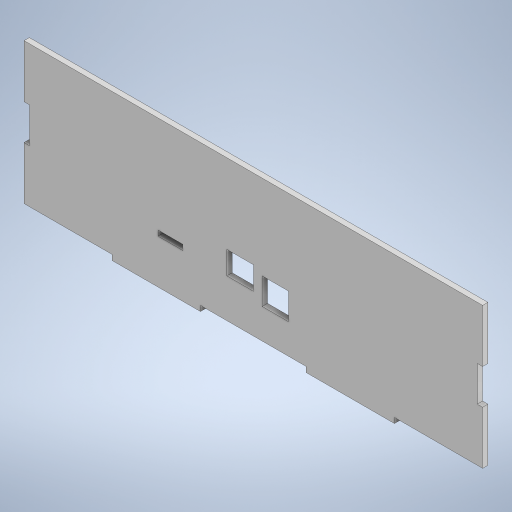
# Autodesk Inventor part: Depan
Saved by Autodesk Inventor 2024 (Build 280153000, 153)
## iProperties
Created: 2023-08-09
Part Number: Depan
Material: Generic
Document SubType Name: Modeling
Designer: Asus
Density: 1 g/cm^3
Appearance: Default
Author: Asus
Autodesk Inventor part; units mm, degrees
ref_plane "YZ Plane" through (0, 0, 0) normal (1, 0, 0) x (0, 1, 0)
ref_plane "XZ Plane" through (0, 0, 0) normal (0, 1, 0) x (-1, 0, 0)
ref_plane "XY Plane" through (0, 0, 0) normal (0, 0, 1) x (1, 0, 0)
sketch "Sketch1" plane through (0, 0, 0) normal (0, 0, 1) x (1, 0, 0)
  line L0 (0, 0) -> (0, 3) construction
  line L1 (0, 3) -> (50, 3)
  line L2 (50, 3) -> (50, 0)
  line L3 (50, 0) -> (100, 0)
  line L4 (100, 0) -> (100, 3)
  line L5 (100, 3) -> (160, 3)
  line L6 (160, 3) -> (160, 0)
  line L7 (160, 0) -> (210, 0)
  line L8 (210, 0) -> (210, 3)
  line L9 (210, 3) -> (260, 3)
  line L10 (260, 3) -> (260, 33)
  line L11 (260, 33) -> (257, 33)
  line L12 (257, 33) -> (257, 53)
  line L13 (257, 53) -> (260, 53)
  line L14 (260, 53) -> (260, 83)
  line L15 (0, 83) -> (0, 53)
  line L16 (0, 53) -> (3, 53)
  line L17 (3, 53) -> (3, 33)
  line L18 (3, 33) -> (0, 33)
  line L19 (0, 33) -> (0, 3)
  line L20 (260, 0) -> (260, 25) construction
  line L21 (260, 25) -> (260, 28) construction
  line L22 (260, 28) -> (90, 28) construction
  line L23 (90, 28) -> (90, 25)
  line L24 (90, 25) -> (76, 25)
  line L25 (76, 25) -> (76, 28)
  line L26 (76, 28) -> (90, 28)
  line L27 (90, 28) -> (135, 28) construction
  line L28 (135, 28) -> (135, 0) construction
  line L29 (135, 0) -> (135, 20) construction
  line L30 (135, 20) -> (150, 20) construction
  line L31 (135, 20) -> (135, 35)
  line L32 (135, 35) -> (150, 35)
  line L33 (150, 35) -> (150, 20)
  line L34 (135, 20) -> (150, 20)
  line L35 (90, 28) -> (117, 28) construction
  line L36 (117, 28) -> (130, 28) construction
  line L37 (130, 28) -> (130, 0) construction
  line L38 (130, 0) -> (130, 25) construction
  line L39 (130, 25) -> (130, 38) construction
  line L40 (130, 25) -> (115, 25)
  line L41 (115, 25) -> (115, 38)
  line L42 (115, 38) -> (130, 38)
  line L43 (130, 25) -> (130, 38)
  line L44 (0, 83) -> (260, 83)
  point P0 (0, 18)
  dimension "d0" = 3
  dimension "d2" = 50
  dimension "d3" = 60
  dimension "d4" = 50
  dimension "d5" = 50
  dimension "d6" = 30
  dimension "d7" = 3
  dimension "d8" = 20
  dimension "d9" = 30
  dimension "d10" = 30
  dimension "d11" = 3
  dimension "d12" = 20
  dimension "d19" = 25
  dimension "d20" = 3
  dimension "d21" = 170
  dimension "d22" = 14
  dimension "d23" = 45
  dimension "d24" = 20
  dimension "d25" = 15
  dimension "d26" = 15
  dimension "d27" = 27
  dimension "d28" = 13
  dimension "d29" = 25
  dimension "d30" = 13
  dimension "d31" = 13
  constraints: 90 end point, 22 point on line, 20 perpendicular, 3 horizontal, 3 vertical, 1 collinear, 1 midpoint
  measures "d0" distance of L0.start L0.end
  measures "d2" distance of L2.end L3.end
  measures "d3" distance of L4.end L5.end
  measures "d4" distance of L6.end L7.end
  measures "d5" distance of L8.end L9.end
  measures "d6" distance of L9.end L10.end
  measures "d7" distance of L10.end L11.end
  measures "d8" distance of L11.end L12.end
  measures "d9" distance of L13.end L14.end
  measures "d10" distance of L15.start L15.end
  measures "d11" distance of L15.end L16.end
  measures "d12" distance of L16.end L17.end
  measures "d19" distance of L20.start L20.end
  measures "d20" distance of L20.end L21.end
  measures "d21" distance of L21.end L22.end
  measures "d22" distance of L23.end L24.end
  measures "d23" distance of L22.end L27.end
  measures "d24" distance of L28.end L29.end
  measures "d25" distance of L29.end L30.end
  measures "d26" distance of L29.end L31.end
  measures "d27" distance of L22.end L35.end
  measures "d28" distance of L35.end L36.end
  measures "d29" distance of L37.end L38.end
  measures "d30" distance of L38.end L39.end
  measures "d31" distance of L40.end L41.end
extrude "Extrusion1" add sketch "Sketch1" along normal blind 3
body "Solid1"
